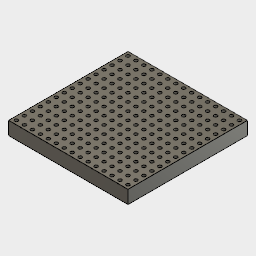
MEC Board (Autodesk Fusion 360 design; units mm, degrees)
Autodesk Fusion 360 part; units mm, degrees
sketch "Sketch1" plane through (0, 0, 0) normal (0, 0, 1) x (1, 0, 0)
  line L0 (-57.15, 57.15) -> (57.15, 57.15)
  line L1 (57.15, 57.15) -> (57.15, -57.15)
  line L2 (57.15, -57.15) -> (-57.15, -57.15)
  line L3 (-57.15, -57.15) -> (-57.15, 57.15)
  line L4 (-57.15, 57.15) -> (57.15, -57.15) construction
  line L5 (57.15, 57.15) -> (-57.15, -57.15) construction
  dimension "d1" = 114.3
  dimension "d2" = 114.3
  constraint perpendicular L0 L1
  constraint parallel L0 L2
  constraint parallel L1 L3
  constraint horizontal L0
  constraint coincident L4 origin
  constraint coincident L5 origin
  measures "d1" distance of L0 L2
  measures "d190" distance of origin
  measures "d193" distance of origin
  measures "d197" distance of origin
extrude "Extrude1" add sketch "Sketch1" along normal blind 12.7
sketch "Sketch2" plane through (0, 0, 12.7) normal (0, 0, 1) x (1, 0, 0)
  line L0 (-57.15, -57.15) -> (57.15, -57.15)
  line L1 (57.15, -57.15) -> (57.15, 57.15)
  line L2 (57.15, 57.15) -> (-57.15, 57.15)
  line L3 (-57.15, 57.15) -> (-57.15, -57.15)
  dimension "d5" = 3.81
  dimension "d6" = 7.62
  dimension "d7" = 3.81
  dimension "d8" = 3.81
  dimension "d9" = 3.81
  dimension "d10" = 7.62
  dimension "d11" = 7.62
  dimension "d12" = 7.62
  dimension "d13" = 7.62
  dimension "d14" = 7.62
  dimension "d15" = 7.62
  dimension "d16" = 7.62
  dimension "d17" = 7.62
  dimension "d18" = 7.62
  dimension "d19" = 3.81
  dimension "d20" = 7.62
  dimension "d21" = 3.81
  dimension "d22" = 3.81
  dimension "d23" = 3.81
  dimension "d24" = 3.81
  dimension "d27" = 7.62
  dimension "d28" = 7.62
  dimension "d29" = 7.62
  dimension "d30" = 3.81
  dimension "d31" = 7.62
  dimension "d32" = 7.62
  dimension "d33" = 7.62
  dimension "d34" = 7.62
  dimension "d35" = 7.62
  dimension "d36" = 7.62
  dimension "d37" = 7.62
  dimension "d38" = 7.62
  dimension "d39" = 7.62
  dimension "d40" = 7.62
  dimension "d41" = 7.62
  dimension "d42" = 7.62
  dimension "d43" = 7.62
  dimension "d44" = 7.62
  dimension "d45" = 7.62
  dimension "d46" = 7.62
  dimension "d47" = 7.62
  dimension "d48" = 7.62
  dimension "d49" = 7.62
  dimension "d50" = 7.62
  dimension "d51" = 7.62
  dimension "d52" = 7.62
  dimension "d53" = 7.62
  dimension "d54" = 7.62
  dimension "d55" = 7.62
  dimension "d56" = 7.62
  dimension "d57" = 7.62
  dimension "d58" = 7.62
  dimension "d59" = 7.62
  dimension "d60" = 7.62
  dimension "d61" = 7.62
  dimension "d62" = 7.62
  dimension "d63" = 7.62
  dimension "d64" = 7.62
  dimension "d65" = 7.62
  dimension "d66" = 7.62
  dimension "d67" = 7.62
  dimension "d68" = 7.62
  dimension "d69" = 7.62
  dimension "d70" = 7.62
  dimension "d71" = 7.62
  dimension "d72" = 7.62
  dimension "d73" = 7.62
  dimension "d74" = 7.62
  dimension "d75" = 7.62
  dimension "d76" = 7.62
  dimension "d77" = 7.62
  dimension "d78" = 7.62
  dimension "d79" = 7.62
  dimension "d80" = 7.62
  dimension "d81" = 7.62
  dimension "d82" = 7.62
  dimension "d83" = 7.62
  dimension "d84" = 7.62
  dimension "d85" = 7.62
  dimension "d86" = 7.62
  dimension "d87" = 7.62
  dimension "d88" = 7.62
  dimension "d89" = 7.62
  dimension "d90" = 7.62
  dimension "d91" = 7.62
  dimension "d92" = 7.62
  dimension "d93" = 7.62
  dimension "d94" = 7.62
  dimension "d95" = 7.62
  dimension "d96" = 7.62
  dimension "d97" = 7.62
  dimension "d98" = 7.62
  dimension "d99" = 7.62
  dimension "d100" = 7.62
  dimension "d101" = 7.62
  dimension "d102" = 7.62
  dimension "d103" = 7.62
  dimension "d104" = 7.62
  dimension "d105" = 7.62
  dimension "d106" = 7.62
  dimension "d107" = 7.62
  dimension "d108" = 7.62
  dimension "d109" = 7.62
  dimension "d110" = 7.62
  dimension "d111" = 7.62
  dimension "d112" = 7.62
  dimension "d113" = 7.62
  dimension "d114" = 7.62
  dimension "d115" = 7.62
  dimension "d116" = 7.62
  dimension "d117" = 7.62
  dimension "d118" = 7.62
  dimension "d119" = 7.62
  dimension "d120" = 7.62
  dimension "d121" = 7.62
  dimension "d122" = 7.62
  dimension "d123" = 7.62
  dimension "d124" = 7.62
  dimension "d125" = 7.62
  dimension "d126" = 7.62
  dimension "d127" = 7.62
  dimension "d128" = 7.62
  dimension "d129" = 7.62
  dimension "d130" = 7.62
  dimension "d131" = 7.62
  dimension "d132" = 7.62
  dimension "d133" = 7.62
  dimension "d134" = 7.62
  dimension "d135" = 7.62
  dimension "d136" = 7.62
  dimension "d137" = 7.62
  dimension "d138" = 7.62
  dimension "d139" = 7.62
  dimension "d140" = 7.62
  dimension "d141" = 7.62
  dimension "d142" = 7.62
  dimension "d143" = 7.62
  dimension "d144" = 7.62
  dimension "d145" = 7.62
  dimension "d146" = 7.62
  dimension "d147" = 7.62
  dimension "d148" = 7.62
  dimension "d149" = 7.62
  dimension "d150" = 7.62
  dimension "d151" = 7.62
  dimension "d152" = 7.62
  dimension "d153" = 7.62
  dimension "d154" = 7.62
  dimension "d155" = 7.62
  dimension "d156" = 7.62
  dimension "d157" = 7.62
  dimension "d158" = 7.62
  dimension "d159" = 7.62
  dimension "d160" = 7.62
  dimension "d161" = 7.62
  dimension "d162" = 7.62
  dimension "d163" = 7.62
  dimension "d164" = 7.62
  dimension "d165" = 7.62
  dimension "d166" = 7.62
  dimension "d167" = 7.62
  dimension "d168" = 7.62
  dimension "d169" = 7.62
  dimension "d170" = 7.62
  dimension "d171" = 7.62
  dimension "d172" = 7.62
  dimension "d173" = 7.62
  dimension "d174" = 7.62
  dimension "d175" = 7.62
  dimension "d176" = 7.62
  dimension "d177" = 7.62
  dimension "d178" = 7.62
  dimension "d179" = 7.62
  dimension "d180" = 7.62
  dimension "d181" = 7.62
  dimension "d182" = 7.62
  dimension "d183" = 7.62
  dimension "d184" = 7.62
  dimension "d185" = 7.62
  dimension "d186" = 7.62
  dimension "d187" = 7.62
  dimension "d188" = 7.62
  dimension "d189" = 7.62
  dimension "d190" = 7.62
  dimension "d191" = 7.62
  dimension "d192" = 7.62
  dimension "d193" = 7.62
  dimension "d194" = 7.62
  dimension "d195" = 7.62
  dimension "d196" = 7.62
  dimension "d197" = 7.62
  dimension "d198" = 7.62
  dimension "d199" = 7.62
  dimension "d200" = 7.62
  dimension "d201" = 7.62
  dimension "d202" = 7.62
  dimension "d203" = 7.62
  dimension "d204" = 7.62
  dimension "d205" = 7.62
  dimension "d206" = 7.62
  dimension "d207" = 7.62
  dimension "d208" = 7.62
  dimension "d209" = 7.62
  dimension "d210" = 7.62
  dimension "d211" = 7.62
  dimension "d212" = 7.62
  dimension "d213" = 7.62
  dimension "d214" = 7.62
  dimension "d215" = 7.62
  dimension "d216" = 7.62
  dimension "d217" = 7.62
  dimension "d218" = 7.62
  dimension "d219" = 7.62
  dimension "d220" = 7.62
  dimension "d221" = 7.62
  dimension "d222" = 7.62
  dimension "d223" = 7.62
  dimension "d224" = 7.62
  dimension "d225" = 7.62
  dimension "d226" = 7.62
  dimension "d227" = 7.62
  dimension "d228" = 7.62
  dimension "d229" = 7.62
  dimension "d230" = 7.62
  dimension "d231" = 7.62
  dimension "d232" = 7.62
  dimension "d233" = 7.62
  dimension "d234" = 7.62
  dimension "d235" = 7.62
  dimension "d236" = 7.62
  dimension "d237" = 7.62
  dimension "d238" = 7.62
  dimension "d239" = 7.62
  dimension "d240" = 7.62
  measures "d5" distance of L3 origin
  measures "d7" distance of L2 origin
  measures "d8" distance of L2 origin
  measures "d9" distance of L2 origin
  measures "d19" distance of L2 origin
  measures "d21" distance of L2 origin
  measures "d22" distance of L2 origin
  measures "d23" distance of L2 origin
  measures "d24" distance of L2 origin
  measures "d30" distance of L1 origin
hole "Hole1" at (-53.34, 53.34, 12.7) at (-45.72, 53.34, 12.7) at (-38.1, 53.34, 12.7) at (-30.48, 53.34, 12.7) at (-22.86, 53.34, 12.7) at (-15.24, 53.34, 12.7) at (-7.62, 53.34, 12.7) at (0, 53.34, 12.7) at (7.62, 53.34, 12.7) at (15.24, 53.34, 12.7) at (22.86, 53.34, 12.7) at (30.48, 53.34, 12.7) at (38.1, 53.34, 12.7) at (45.72, 53.34, 12.7) at (53.34, 53.34, 12.7) at (-15.24, 15.24, 12.7) at (-15.24, 22.86, 12.7) at (-45.72, 15.24, 12.7) at (-53.34, 38.1, 12.7) at (-7.62, 15.24, 12.7) at (45.72, 30.48, 12.7) at (-22.86, 15.24, 12.7) at (0, 38.1, 12.7) at (-7.62, 0, 12.7) at (-45.72, 7.62, 12.7) at (-7.62, 7.62, 12.7) at (15.24, 15.24, 12.7) at (-30.48, 15.24, 12.7) at (7.62, 15.24, 12.7) at (-38.1, 15.24, 12.7) at (-15.24, 7.62, 12.7) at (15.24, 22.86, 12.7) at (-30.48, 22.86, 12.7) at (-45.72, 0, 12.7) at (-22.86, 7.62, 12.7) at (7.62, 22.86, 12.7) at (-15.24, 0, 12.7) at (-22.86, 0, 12.7) at (-38.1, 22.86, 12.7) at (53.34, -15.24, 12.7) at (7.62, 0, 12.7) at (30.48, -15.24, 12.7) at (0, 15.24, 12.7) at (0, 7.62, 12.7) at (-38.1, 0, 12.7) at (-53.34, 15.24, 12.7) at (0, 0, 12.7) at (-53.34, 22.86, 12.7) at (-53.34, 7.62, 12.7) at (-53.34, 0, 12.7) at (0, 22.86, 12.7) at (-15.24, -7.62, 12.7) at (15.24, 0, 12.7) at (38.1, -15.24, 12.7) at (-7.62, -15.24, 12.7) at (15.24, -15.24, 12.7) at (22.86, -15.24, 12.7) at (-38.1, -15.24, 12.7) at (-53.34, -38.1, 12.7) at (-53.34, -53.34, 12.7) at (0, -38.1, 12.7) at (0, -45.72, 12.7) at (-53.34, -45.72, 12.7) at (-53.34, -15.24, 12.7) at (22.86, -45.72, 12.7) at (7.62, -15.24, 12.7) at (45.72, -45.72, 12.7) at (0, -15.24, 12.7) at (-38.1, -45.72, 12.7) at (45.72, -15.24, 12.7) at (0, -53.34, 12.7) at (-30.48, -53.34, 12.7) at (22.86, -53.34, 12.7) at (7.62, -53.34, 12.7) at (-22.86, -38.1, 12.7) at (-45.72, -45.72, 12.7) at (-45.72, -38.1, 12.7) at (30.48, -45.72, 12.7) at (53.34, -38.1, 12.7) at (-15.24, -45.72, 12.7) at (15.24, -53.34, 12.7) at (38.1, -38.1, 12.7) at (30.48, -38.1, 12.7) at (-38.1, -53.34, 12.7) at (-22.86, -45.72, 12.7) at (45.72, -53.34, 12.7) at (-15.24, -22.86, 12.7) at (38.1, -22.86, 12.7) at (-7.62, -30.48, 12.7) at (30.48, -22.86, 12.7) at (-7.62, -22.86, 12.7) at (-30.48, -15.24, 12.7) at (53.34, -22.86, 12.7) at (30.48, -30.48, 12.7) at (-22.86, -22.86, 12.7) at (-45.72, -30.48, 12.7) at (-15.24, -30.48, 12.7) at (53.34, -30.48, 12.7) at (-22.86, -30.48, 12.7) at (-45.72, -22.86, 12.7) at (38.1, -30.48, 12.7) at (-30.48, -7.62, 12.7) at (-7.62, 38.1, 12.7) at (7.62, 38.1, 12.7) at (-30.48, 38.1, 12.7) at (15.24, 38.1, 12.7) at (-22.86, 38.1, 12.7) at (38.1, 38.1, 12.7) at (22.86, 38.1, 12.7) at (-38.1, 38.1, 12.7) at (7.62, 45.72, 12.7) at (45.72, 45.72, 12.7) at (-30.48, 45.72, 12.7) at (22.86, 45.72, 12.7) at (15.24, 45.72, 12.7) at (0, 45.72, 12.7) at (38.1, 30.48, 12.7) at (-15.24, 38.1, 12.7) at (-45.72, 22.86, 12.7) at (-38.1, 7.62, 12.7) at (-7.62, 22.86, 12.7) at (7.62, 7.62, 12.7) at (15.24, 7.62, 12.7) at (-30.48, 7.62, 12.7) at (-30.48, 0, 12.7) at (-22.86, 22.86, 12.7) at (22.86, 30.48, 12.7) at (7.62, 30.48, 12.7) at (-53.34, 30.48, 12.7) at (0, 30.48, 12.7) at (45.72, 38.1, 12.7) at (-30.48, 30.48, 12.7) at (15.24, 30.48, 12.7) at (-38.1, 30.48, 12.7) at (-22.86, -15.24, 12.7) at (-45.72, -15.24, 12.7) at (-45.72, -7.62, 12.7) at (15.24, -22.86, 12.7) at (-38.1, -22.86, 12.7) at (-38.1, -7.62, 12.7) at (22.86, -22.86, 12.7) at (7.62, -7.62, 12.7) at (15.24, -7.62, 12.7) at (-30.48, -22.86, 12.7) at (45.72, -22.86, 12.7) at (-15.24, -15.24, 12.7) at (-22.86, -7.62, 12.7) at (-30.48, -30.48, 12.7) at (-7.62, -7.62, 12.7) at (7.62, -22.86, 12.7) at (-45.72, 30.48, 12.7) at (-15.24, 30.48, 12.7) at (-53.34, 45.72, 12.7) at (-45.72, 38.1, 12.7) at (30.48, 30.48, 12.7) at (30.48, 38.1, 12.7) at (-7.62, 30.48, 12.7) at (-22.86, 30.48, 12.7) at (0, -22.86, 12.7) at (15.24, -30.48, 12.7) at (-30.48, -38.1, 12.7) at (-7.62, -53.34, 12.7) at (15.24, -38.1, 12.7) at (-15.24, -53.34, 12.7) at (0, -30.48, 12.7) at (53.34, -53.34, 12.7) at (7.62, -38.1, 12.7) at (7.62, -30.48, 12.7) at (-38.1, -30.48, 12.7) at (22.86, -38.1, 12.7) at (30.48, -53.34, 12.7) at (-53.34, -7.62, 12.7) at (22.86, -30.48, 12.7) at (15.24, -45.72, 12.7) at (-53.34, -30.48, 12.7) at (45.72, -30.48, 12.7) at (-38.1, -38.1, 12.7) at (0, -7.62, 12.7) at (-22.86, -53.34, 12.7) at (38.1, -53.34, 12.7) at (-15.24, -38.1, 12.7) at (38.1, -45.72, 12.7) at (7.62, -45.72, 12.7) at (-7.62, -38.1, 12.7) at (-7.62, -45.72, 12.7) at (53.34, -45.72, 12.7) at (45.72, -38.1, 12.7) at (-53.34, -22.86, 12.7) at (-45.72, -53.34, 12.7) at (-30.48, -45.72, 12.7) at (0, 0, 12.7) at (30.48, 45.72, 12.7) at (-7.62, 45.72, 12.7) at (-38.1, 45.72, 12.7) at (38.1, 45.72, 12.7) at (-15.24, 45.72, 12.7) at (-45.72, 45.72, 12.7) at (-22.86, 45.72, 12.7) at (30.48, 0, 12.7) at (22.86, 15.24, 12.7) at (45.72, 0, 12.7) at (22.86, 0, 12.7) at (38.1, 0, 12.7) at (38.1, 7.62, 12.7) at (45.72, 15.24, 12.7) at (30.48, 7.62, 12.7) at (45.72, 7.62, 12.7) at (38.1, 15.24, 12.7) at (30.48, 15.24, 12.7) at (22.86, 7.62, 12.7) at (53.34, 38.1, 12.7) at (53.34, 45.72, 12.7) at (53.34, 30.48, 12.7) at (53.34, 22.86, 12.7) at (45.72, 22.86, 12.7) at (38.1, 22.86, 12.7) at (30.48, 22.86, 12.7) at (22.86, 22.86, 12.7) at (22.86, -7.62, 12.7) at (30.48, -7.62, 12.7) at (38.1, -7.62, 12.7) at (45.72, -7.62, 12.7) at (53.34, -7.62, 12.7) at (53.34, 0, 12.7) at (53.34, 7.62, 12.7) at (53.34, 15.24, 12.7) direction (0, 0, -1) diameter 3.175 end through all
move_body "MoveBody1" bodies 1 to x (1, 0, 0) y (0, 0, -1) z (0, 1, 0) at (0, 57.15, 57.15)
